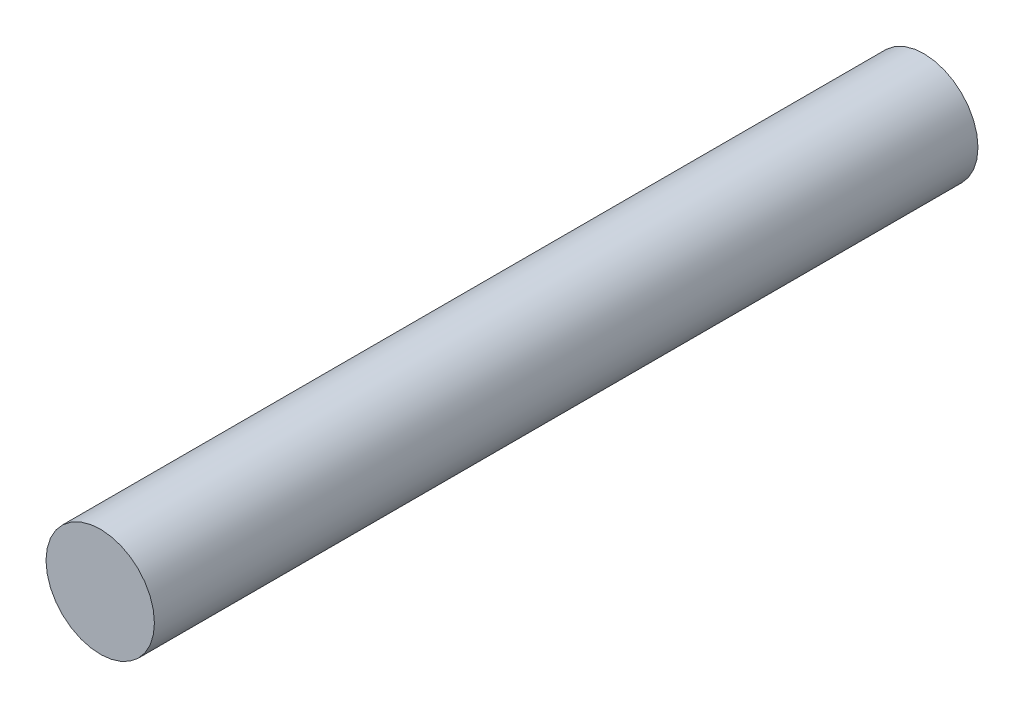
# Autodesk Inventor part: handle_holder
Saved by Autodesk Inventor 2021 (Build 250183000, 183)
## iProperties
Created: 2021-07-05
Part Number: handle_holder
Material: Generic
Document SubType Name: Modeling
Designer: teh18
Density: 1 g/cm^3
Appearance: Default
Author: teh18
Autodesk Inventor part; units mm, degrees
ref_plane "YZ Plane" through (0, 0, 0) normal (1, 0, 0) x (0, 1, 0)
ref_plane "XZ Plane" through (0, 0, 0) normal (0, 1, 0) x (-1, 0, 0)
ref_plane "XY Plane" through (0, 0, 0) normal (0, 0, 1) x (1, 0, 0)
sketch "Sketch1" plane through (0, 0, 0) normal (0, 0, 1) x (1, 0, 0)
  spline S0 degree 3 poles (4.05, 0) (4.05, -0.5086) (3.9482, -1.0443) (3.5509, -2.0173) (3.256, -2.4551) (2.5583, -3.1847) (2.0935, -3.5108) (1.0757, -3.9435) (0.5224, -4.05) (-0.5016, -4.05) (-1.045, -3.9511) (-2.0577, -3.5311) (-2.5267, -3.2096) (-3.2421, -2.4765) (-3.5453, -2.0291) (-3.9493, -1.0437) (-4.05, -0.5057) (-4.05, 0.5057) (-3.9493, 1.0437) (-3.5453, 2.0291) (-3.2421, 2.4765) (-2.5267, 3.2096) (-2.0577, 3.5311) (-1.045, 3.9511) (-0.5016, 4.05) (0.5224, 4.05) (1.0757, 3.9435) (2.0935, 3.5108) (2.5583, 3.1847) (3.256, 2.4551) (3.5509, 2.0173) (3.9482, 1.0443) (4.05, 0.5086) (4.05, 0) knots 0 0 0 0 0.152581 0.152581 0.305163 0.305163 0.476115 0.476115 0.647066 0.647066 0.81122 0.81122 0.975373 0.975373 1.12709 1.12709 1.278806 1.278806 1.430523 1.430523 1.58224 1.58224 1.746393 1.746393 1.910546 1.910546 2.081498 2.081498 2.25245 2.25245 2.405031 2.405031 2.557613 2.557613 2.557613 2.557613 projected
  spline S1 degree 5 poles (3.95, 0) (3.9504, -0.3667) (3.9036, -0.7326) (3.8228, -1.0932) (3.577, -1.7696) (3.1848, -2.371) (2.9667, -2.6454) (2.4667, -3.1307) (1.8774, -3.5003) (1.5647, -3.6531) (0.9169, -3.8771) (0.2376, -3.9646) (-0.1023, -3.9714) (-0.7953, -3.9042) (-1.4604, -3.6977) (-1.7879, -3.549) (-2.4046, -3.1805) (-2.9304, -2.6887) (-3.1591, -2.4073) (-3.5658, -1.7963) (-3.8198, -1.1054) (-3.9029, -0.7414) (-3.9972, 0) (-3.9029, 0.7414) (-3.8198, 1.1054) (-3.5658, 1.7963) (-3.1591, 2.4073) (-2.9304, 2.6887) (-2.4046, 3.1805) (-1.7879, 3.549) (-1.4604, 3.6977) (-0.7953, 3.9042) (-0.1023, 3.9714) (0.2376, 3.9646) (0.9169, 3.8771) (1.5647, 3.6531) (1.8774, 3.5003) (2.4667, 3.1307) (2.9667, 2.6454) (3.1848, 2.371) (3.577, 1.7696) (3.8228, 1.0932) (3.9036, 0.7326) (3.9504, 0.3667) (3.95, 0) knots 0 0 0 0 0 0 0.07386 0.07386 0.07386 0.143894 0.143894 0.143894 0.213351 0.213351 0.213351 0.281227 0.281227 0.281227 0.35291 0.35291 0.35291 0.425292 0.425292 0.425292 0.5 0.5 0.5 0.574708 0.574708 0.574708 0.64709 0.64709 0.64709 0.718773 0.718773 0.718773 0.786649 0.786649 0.786649 0.856106 0.856106 0.856106 0.92614 0.92614 0.92614 1 1 1 1 1 1
  point P0 (0, 0)
  point P1 (4.05, 0)
  dimension "d2" = 0.1
  constraints: 2 other
extrude "Extrusion1" add sketch "Sketch1" along normal mid plane 60 contours S1
body "Solid1"
